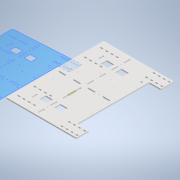
# Autodesk Inventor part: Korpus 3
Saved by Autodesk Inventor 2021.1 (Build 251245010, 245A)
## iProperties
Created: 2023-03-13
Part Number: Korpus 3
Material: Типовые
Document SubType Name: Modeling
Designer: User
Density: 1 g/cm^3
Appearance: По умолчанию
Author: User
Autodesk Inventor part; units mm, degrees
ref_plane "YZ Plane" through (0, 0, 0) normal (1, 0, 0) x (0, 1, 0)
ref_plane "XZ Plane" through (0, 0, 0) normal (0, 1, 0) x (-1, 0, 0)
ref_plane "XY Plane" through (0, 0, 0) normal (0, 0, 1) x (1, 0, 0)
ref_plane "РабПлоскость1" through (117.6762, -49.065, -12.9978) normal (0, -1, 0) x (1, 0, 0)
sketch "Эскиз2" plane through (117.6762, -49.065, -12.9978) normal (0, -1, 0) x (1, 0, 0)
  line L0 (-0.1, 156.35) -> (-0.1, 125.1) projected
  line L1 (-0.1, 125.1) -> (6.1, 125.1) projected
  line L2 (6.1, 156.35) -> (6.1, 125.1) projected
  line L3 (-0.1, 156.35) -> (6.1, 156.35) projected
  line L4 (-0.1, 93.85) -> (-0.1, 62.6) projected
  line L5 (-0.1, 62.6) -> (6.1, 62.6) projected
  line L6 (6.1, 93.85) -> (6.1, 62.6) projected
  line L7 (-0.1, 93.85) -> (6.1, 93.85) projected
  line L8 (-0.1, 31.35) -> (-0.1, 0.1) projected
  line L9 (-0.1, 0.1) -> (6.1, 0.1) projected
  line L10 (6.1, 31.35) -> (6.1, 0.1) projected
  line L11 (-0.1, 31.35) -> (6.1, 31.35) projected
  line L12 (-0.1, -31.15) -> (-0.1, -62.4) projected
  line L13 (-0.1, -62.4) -> (6.1, -62.4) projected
  line L14 (6.1, -31.15) -> (6.1, -62.4) projected
  line L15 (-0.1, -31.15) -> (6.1, -31.15) projected
  line L16 (-0.1, -93.65) -> (-0.1, -124.9) projected
  line L17 (-0.1, -124.9) -> (6.1, -124.9) projected
  line L18 (6.1, -93.65) -> (6.1, -124.9) projected
  line L19 (-0.1, -93.65) -> (6.1, -93.65) projected
  line L20 (-0.1, -156.15) -> (-0.1, -187.4) projected
  line L21 (-0.1, -187.4) -> (6.1, -187.4) projected
  line L22 (6.1, -156.15) -> (6.1, -187.4) projected
  line L23 (-0.1, -156.15) -> (6.1, -156.15) projected
  line L24 (-0.1, -218.65) -> (-0.1, -249.9) projected
  line L25 (-0.1, -249.9) -> (6.1, -249.9) projected
  line L26 (6.1, -218.65) -> (6.1, -249.9) projected
  line L27 (-0.1, -218.65) -> (6.1, -218.65) projected
  line L28 (-0.1, -281.15) -> (-0.1, -312.4) projected
  line L29 (-0.1, -312.4) -> (6.1, -312.4) projected
  line L30 (6.1, -281.15) -> (6.1, -312.4) projected
  line L31 (-0.1, -281.15) -> (6.1, -281.15) projected
  line L32 (21.75, -81.125) -> (59.25, -81.125) projected
  line L33 (59.25, -81.125) -> (59.25, -74.925) projected
  line L34 (21.75, -74.925) -> (59.25, -74.925) projected
  line L35 (21.75, -81.125) -> (21.75, -74.925) projected
  line L36 (96.75, -81.125) -> (134.25, -81.125) projected
  line L37 (134.25, -81.125) -> (134.25, -74.925) projected
  line L38 (96.75, -74.925) -> (134.25, -74.925) projected
  line L39 (96.75, -81.125) -> (96.75, -74.925) projected
  line L40 (-53.25, -81.125) -> (-15.75, -81.125) projected
  line L41 (-15.75, -81.125) -> (-15.75, -74.925) projected
  line L42 (-53.25, -74.925) -> (-15.75, -74.925) projected
  line L43 (-53.25, -81.125) -> (-53.25, -74.925) projected
  line L44 (-128.25, -81.125) -> (-90.75, -81.125) projected
  line L45 (-90.75, -81.125) -> (-90.75, -74.925) projected
  line L46 (-128.25, -74.925) -> (-90.75, -74.925) projected
  line L47 (-128.25, -81.125) -> (-128.25, -74.925) projected
  line L48 (-0.1, -328.025) -> (6.1, -328.025) construction
  line L49 (-147, -81.125) -> (-147, -74.925) construction
  line L50 (-0.1, 171.975) -> (6.1, 171.975) construction
  line L51 (153, -81.125) -> (153, -74.925) construction
  line L52 (208, 171.975) -> (-142, 171.975)
  line L53 (-142, -328.025) -> (208, -328.025)
  line L54 (153, -256.225) -> (153, 100.175)
  line L55 (158, 105.175) -> (208, 105.175)
  line L56 (213, 110.175) -> (213, 166.975)
  line L57 (158, -261.225) -> (208, -261.225)
  line L58 (213, -266.225) -> (213, -323.025)
  arc A0 (213, 166.975) -> (208, 171.975) centre (208, 166.975) ccw
  arc A1 (208, 105.175) -> (213, 110.175) centre (208, 110.175) ccw
  arc A2 (158, 105.175) -> (153, 100.175) centre (158, 100.175) ccw
  arc A3 (153, -256.225) -> (158, -261.225) centre (158, -256.225) ccw
  arc A4 (213, -266.225) -> (208, -261.225) centre (208, -266.225) ccw
  arc A5 (208, -328.025) -> (213, -323.025) centre (208, -323.025) ccw
  line L59 (-147, 166.975) -> (-147, -323.025)
  arc A6 (-142, 171.975) -> (-147, 166.975) centre (-142, 166.975) ccw
  arc A7 (-147, -323.025) -> (-142, -328.025) centre (-142, -323.025) ccw
  point P0 (-117.6762, 12.9978)
  point P1 (153, -78.025)
  point P2 (213, -328.025)
  point P3 (153, -261.225)
  point P4 (-147, -328.025)
  point P5 (-147, 171.975)
  point P6 (153, 105.175)
  point P7 (213, 171.975)
  point P8 (213, 105.175)
  point P9 (213, -261.225)
  point P10 (-147, -78.025)
  point P11 (3, 171.975)
  point P12 (3, -328.025)
  dimension "d5" = 6.2
  dimension "d11" = 60
  dimension "d12" = 66.8
  dimension "d14" = 5
  dimension "d15" = 5
  constraints: 19 point on line, 16 end point, 16 point on circle, 16 tangent, 8 centre point, 6 equal radius, 6 midpoint, 4 perpendicular, 3 horizontal, 1 vertical, 1 vertical alignment
  measures "d5" distance between parallel lines of L34 L32
  measures "d11" distance from line of point (213, 171.975) L54
  measures "d12" distance from line of point (153, 105.175) L52
  measures "d14" radius of A0
  measures "d15" radius of A6
extrude "Корпус" add sketch "Эскиз2" along normal blind 6.2
sketch "Эскиз3" plane through (117.6762, -55.265, -12.9978) normal (0, -1, 0) x (1, 0, 0)
  line L0 (-0.1, -281.15) -> (-0.1, -312.4) construction
  line L1 (-0.1, -312.4) -> (6.1, -312.4) construction
  line L2 (6.1, -281.15) -> (6.1, -312.4) construction
  line L3 (-0.1, -281.15) -> (6.1, -281.15) construction
  line L4 (-0.1, -218.65) -> (-0.1, -249.9) construction
  line L5 (-0.1, -249.9) -> (6.1, -249.9) construction
  line L6 (6.1, -218.65) -> (6.1, -249.9) construction
  line L7 (-0.1, -218.65) -> (6.1, -218.65) construction
  line L8 (-0.1, -156.15) -> (-0.1, -187.4) construction
  line L9 (-0.1, -187.4) -> (6.1, -187.4) construction
  line L10 (6.1, -156.15) -> (6.1, -187.4) construction
  line L11 (-0.1, -156.15) -> (6.1, -156.15) construction
  line L12 (-0.1, -93.65) -> (-0.1, -124.9) construction
  line L13 (-0.1, -124.9) -> (6.1, -124.9) construction
  line L14 (6.1, -93.65) -> (6.1, -124.9) construction
  line L15 (-0.1, -93.65) -> (6.1, -93.65) construction
  line L16 (-0.1, -31.15) -> (-0.1, -62.4) construction
  line L17 (-0.1, -62.4) -> (6.1, -62.4) construction
  line L18 (6.1, -31.15) -> (6.1, -62.4) construction
  line L19 (-0.1, -31.15) -> (6.1, -31.15) construction
  line L20 (-0.1, 31.35) -> (-0.1, 0.1) construction
  line L21 (-0.1, 0.1) -> (6.1, 0.1) construction
  line L22 (6.1, 31.35) -> (6.1, 0.1) construction
  line L23 (-0.1, 31.35) -> (6.1, 31.35) construction
  line L24 (-0.1, 93.85) -> (-0.1, 62.6) construction
  line L25 (-0.1, 62.6) -> (6.1, 62.6) construction
  line L26 (6.1, 93.85) -> (6.1, 62.6) construction
  line L27 (-0.1, 93.85) -> (6.1, 93.85) construction
  line L28 (-0.1, 156.35) -> (-0.1, 125.1) construction
  line L29 (-0.1, 125.1) -> (6.1, 125.1) construction
  line L30 (6.1, 156.35) -> (6.1, 125.1) construction
  line L31 (-0.1, 156.35) -> (6.1, 156.35) construction
  line L32 (21.75, -81.125) -> (59.25, -81.125) construction
  line L33 (59.25, -81.125) -> (59.25, -74.925) construction
  line L34 (21.75, -74.925) -> (59.25, -74.925) construction
  line L35 (21.75, -81.125) -> (21.75, -74.925) construction
  line L36 (96.75, -81.125) -> (134.25, -81.125) construction
  line L37 (134.25, -81.125) -> (134.25, -74.925) construction
  line L38 (96.75, -74.925) -> (134.25, -74.925) construction
  line L39 (96.75, -81.125) -> (96.75, -74.925) construction
  line L40 (-53.25, -81.125) -> (-15.75, -81.125) construction
  line L41 (-15.75, -81.125) -> (-15.75, -74.925) construction
  line L42 (-53.25, -74.925) -> (-15.75, -74.925) construction
  line L43 (-53.25, -81.125) -> (-53.25, -74.925) construction
  line L44 (-128.25, -81.125) -> (-90.75, -81.125) construction
  line L45 (-90.75, -81.125) -> (-90.75, -74.925) construction
  line L46 (-128.25, -74.925) -> (-90.75, -74.925) construction
  line L47 (-128.25, -81.125) -> (-128.25, -74.925) construction
  line L48 (-53.25, -81.125) -> (-90.75, -74.925) construction
  line L49 (96.75, -74.925) -> (134.25, -74.925) construction
  line L50 (59.25, -81.125) -> (96.75, -74.925) construction
  line L51 (6.1, -249.9) -> (-0.1, -249.9) construction
  line L52 (6.1, -281.15) -> (-0.1, -249.9) construction
  line L53 (6.1, -218.65) -> (6.1, -249.9) construction
  line L54 (6.1, -187.4) -> (-0.1, -187.4) construction
  line L55 (6.1, -218.65) -> (-0.1, -187.4) construction
  line L56 (6.1, -156.15) -> (6.1, -187.4) construction
  line L57 (6.1, -156.15) -> (-0.1, -124.9) construction
  line L58 (6.1, -62.4) -> (-0.1, -62.4) construction
  line L59 (6.1, -31.15) -> (6.1, -62.4) construction
  line L60 (6.1, -31.15) -> (-0.1, 0.1) construction
  line L61 (6.1, 31.35) -> (-0.1, 62.6) construction
  line L62 (6.1, 93.85) -> (-0.1, 125.1) construction
  circle A0 centre (3, -265.525) radius 2
  circle A1 centre (3, -140.525) radius 2
  circle A2 centre (3, -15.525) radius 2
  circle A3 centre (3, 109.475) radius 2
  circle A4 centre (-72, -78.025) radius 2
  circle A5 centre (78, -78.025) radius 2
  point P0 (-117.6762, 12.9978)
  dimension "d8" = 4
  constraints: 16 end point, 6 centre point, 6 midpoint, 5 equal radius, 2 parallel
  measures "d8" diameter of A4
extrude "Отверстия" cut sketch "Эскиз3" against normal blind 6.2
sketch "Эскиз6" plane through (117.6762, -55.265, -12.9978) normal (0, -1, 0) x (1, 0, 0)
  line L0 (208, 171.975) -> (-142, 171.975) construction
  line L1 (213, 110.175) -> (213, 166.975) construction
  line L2 (158, 105.175) -> (208, 105.175) construction
  line L3 (-147, 166.975) -> (-147, -323.025) construction
  line L4 (195.1429, 160.775) -> (208, 160.775)
  line L5 (208, 160.775) -> (208, 154.575)
  line L6 (208, 154.575) -> (195.1429, 154.575)
  line L7 (195.1429, 154.575) -> (195.1429, 160.775)
  line L8 (195.1429, 122.575) -> (208, 122.575)
  line L9 (208, 122.575) -> (208, 116.375)
  line L10 (208, 116.375) -> (195.1429, 116.375)
  line L11 (195.1429, 116.375) -> (195.1429, 122.575)
  line L12 (195.1429, 160.775) -> (195.1429, 171.975) construction
  line L13 (195.1429, 116.375) -> (195.1429, 105.175) construction
  line L14 (169.4286, 116.375) -> (169.4286, 122.575)
  line L15 (169.4286, 122.575) -> (182.2857, 122.575)
  line L16 (182.2857, 154.575) -> (169.4286, 154.575)
  line L17 (182.2857, 116.375) -> (169.4286, 116.375)
  line L18 (182.2857, 160.775) -> (182.2857, 154.575)
  line L19 (169.4286, 154.575) -> (169.4286, 160.775)
  line L20 (169.4286, 160.775) -> (182.2857, 160.775)
  line L21 (182.2857, 122.575) -> (182.2857, 116.375)
  line L22 (143.7143, 116.375) -> (143.7143, 122.575)
  line L23 (143.7143, 122.575) -> (156.5714, 122.575)
  line L24 (156.5714, 154.575) -> (143.7143, 154.575)
  line L25 (156.5714, 116.375) -> (143.7143, 116.375)
  line L26 (156.5714, 160.775) -> (156.5714, 154.575)
  line L27 (143.7143, 154.575) -> (143.7143, 160.775)
  line L28 (143.7143, 160.775) -> (156.5714, 160.775)
  line L29 (156.5714, 122.575) -> (156.5714, 116.375)
  line L30 (118, 116.375) -> (118, 122.575)
  line L31 (118, 122.575) -> (130.8571, 122.575)
  line L32 (130.8571, 154.575) -> (118, 154.575)
  line L33 (130.8571, 116.375) -> (118, 116.375)
  line L34 (130.8571, 160.775) -> (130.8571, 154.575)
  line L35 (118, 154.575) -> (118, 160.775)
  line L36 (118, 160.775) -> (130.8571, 160.775)
  line L37 (130.8571, 122.575) -> (130.8571, 116.375)
  line L38 (0, 93.85) -> (0, 62.6) construction
  line L39 (-0.1, 62.5) -> (6.1, 62.5) construction
  line L40 (6, 93.85) -> (6, 62.6) construction
  line L41 (-0.1, 93.75) -> (6.1, 93.75) construction
  line L42 (-53.25, -81.125) -> (-15.75, -81.125) construction
  line L43 (-15.75, -81.125) -> (-15.75, -74.925) construction
  line L44 (-53.25, -74.925) -> (-15.75, -74.925) construction
  line L45 (-53.25, -81.125) -> (-53.25, -74.925) construction
  line L46 (21.75, -81.125) -> (59.25, -81.125) construction
  line L47 (59.25, -81.125) -> (59.25, -74.925) construction
  line L48 (21.75, -74.925) -> (59.25, -74.925) construction
  line L49 (21.75, -81.125) -> (21.75, -74.925) construction
  line L50 (-15.75, -78.025) -> (21.75, -78.025) construction
  line L51 (-127, 137.075) -> (-113.7143, 137.075)
  line L52 (-113.7143, 137.075) -> (-113.7143, 130.875)
  line L53 (-113.7143, 130.875) -> (-127, 130.875)
  line L54 (-127, 130.875) -> (-127, 137.075)
  line L55 (-127, 54.075) -> (-113.7143, 54.075)
  line L56 (-113.7143, 54.075) -> (-113.7143, 47.875)
  line L57 (-113.7143, 47.875) -> (-127, 47.875)
  line L58 (-127, 47.875) -> (-127, 54.075)
  line L59 (-100.4286, 54.075) -> (-87.1429, 54.075)
  line L60 (-87.1429, 47.875) -> (-100.4286, 47.875)
  line L61 (-100.4286, 47.875) -> (-100.4286, 54.075)
  line L62 (-87.1429, 137.075) -> (-87.1429, 130.875)
  line L63 (-87.1429, 130.875) -> (-100.4286, 130.875)
  line L64 (-100.4286, 137.075) -> (-87.1429, 137.075)
  line L65 (-100.4286, 130.875) -> (-100.4286, 137.075)
  line L66 (-87.1429, 54.075) -> (-87.1429, 47.875)
  line L67 (-73.8571, 54.075) -> (-60.5714, 54.075)
  line L68 (-60.5714, 47.875) -> (-73.8571, 47.875)
  line L69 (-73.8571, 47.875) -> (-73.8571, 54.075)
  line L70 (-60.5714, 137.075) -> (-60.5714, 130.875)
  line L71 (-60.5714, 130.875) -> (-73.8571, 130.875)
  line L72 (-73.8571, 137.075) -> (-60.5714, 137.075)
  line L73 (-73.8571, 130.875) -> (-73.8571, 137.075)
  line L74 (-60.5714, 54.075) -> (-60.5714, 47.875)
  line L75 (-47.2857, 54.075) -> (-34, 54.075)
  line L76 (-34, 47.875) -> (-47.2857, 47.875)
  line L77 (-47.2857, 47.875) -> (-47.2857, 54.075)
  line L78 (-34, 137.075) -> (-34, 130.875)
  line L79 (-34, 130.875) -> (-47.2857, 130.875)
  line L80 (-47.2857, 137.075) -> (-34, 137.075)
  line L81 (-47.2857, 130.875) -> (-47.2857, 137.075)
  line L82 (-34, 54.075) -> (-34, 47.875)
  line L83 (-15.75, 93.85) -> (-53.25, 93.85)
  line L84 (-53.25, 93.85) -> (-53.25, 62.6)
  line L85 (-53.25, 62.6) -> (-15.75, 62.6)
  line L86 (-15.75, 62.6) -> (-15.75, 93.85)
  line L87 (21.75, 62.6) -> (59.25, 62.6)
  line L88 (59.25, 62.6) -> (59.25, 93.85)
  line L89 (59.25, 93.85) -> (21.75, 93.85)
  line L90 (21.75, 93.85) -> (21.75, 62.6)
  line L91 (-113.7143, 130.875) -> (-100.4286, 137.075) construction
  line L92 (-60.5714, 130.875) -> (-47.2857, 137.075) construction
  line L93 (-113.7143, 47.875) -> (-100.4286, 54.075) construction
  line L94 (-60.5714, 47.875) -> (-47.2857, 54.075) construction
  line L95 (130.8571, 154.575) -> (143.7143, 160.775) construction
  line L96 (182.2857, 154.575) -> (195.1429, 160.775) construction
  line L97 (130.8571, 116.375) -> (143.7143, 122.575) construction
  line L98 (182.2857, 116.375) -> (195.1429, 122.575) construction
  circle A0 centre (-107.0714, 133.975) radius 1.5
  circle A1 centre (-53.9286, 133.975) radius 1.5
  circle A2 centre (-107.0714, 50.975) radius 1.5
  circle A3 centre (-53.9286, 50.975) radius 1.5
  circle A4 centre (137.2857, 157.675) radius 1.5
  circle A5 centre (188.7143, 157.675) radius 1.5
  circle A6 centre (188.7143, 119.475) radius 1.5
  circle A7 centre (137.2857, 119.475) radius 1.5
  line L99 (195.1429, -316.825) -> (208, -316.825)
  line L100 (208, -316.825) -> (208, -310.625)
  line L101 (208, -310.625) -> (195.1429, -310.625)
  line L102 (195.1429, -310.625) -> (195.1429, -316.825)
  line L103 (195.1429, -278.625) -> (208, -278.625)
  line L104 (208, -278.625) -> (208, -272.425)
  line L105 (208, -272.425) -> (195.1429, -272.425)
  line L106 (195.1429, -272.425) -> (195.1429, -278.625)
  line L107 (195.1429, -316.825) -> (195.1429, -328.025) construction
  line L108 (169.4286, -272.425) -> (169.4286, -278.625)
  line L109 (169.4286, -278.625) -> (182.2857, -278.625)
  line L110 (182.2857, -310.625) -> (169.4286, -310.625)
  line L111 (182.2857, -272.425) -> (169.4286, -272.425)
  line L112 (182.2857, -316.825) -> (182.2857, -310.625)
  line L113 (169.4286, -310.625) -> (169.4286, -316.825)
  line L114 (169.4286, -316.825) -> (182.2857, -316.825)
  line L115 (182.2857, -278.625) -> (182.2857, -272.425)
  line L116 (143.7143, -272.425) -> (143.7143, -278.625)
  line L117 (143.7143, -278.625) -> (156.5714, -278.625)
  line L118 (156.5714, -310.625) -> (143.7143, -310.625)
  line L119 (156.5714, -272.425) -> (143.7143, -272.425)
  line L120 (156.5714, -316.825) -> (156.5714, -310.625)
  line L121 (143.7143, -310.625) -> (143.7143, -316.825)
  line L122 (143.7143, -316.825) -> (156.5714, -316.825)
  line L123 (156.5714, -278.625) -> (156.5714, -272.425)
  line L124 (118, -272.425) -> (118, -278.625)
  line L125 (118, -278.625) -> (130.8571, -278.625)
  line L126 (130.8571, -310.625) -> (118, -310.625)
  line L127 (130.8571, -272.425) -> (118, -272.425)
  line L128 (130.8571, -316.825) -> (130.8571, -310.625)
  line L129 (118, -310.625) -> (118, -316.825)
  line L130 (118, -316.825) -> (130.8571, -316.825)
  line L131 (130.8571, -278.625) -> (130.8571, -272.425)
  line L132 (130.8571, -310.625) -> (143.7143, -316.825) construction
  line L133 (182.2857, -310.625) -> (195.1429, -316.825) construction
  line L134 (130.8571, -272.425) -> (143.7143, -278.625) construction
  line L135 (182.2857, -272.425) -> (195.1429, -278.625) construction
  circle A8 centre (137.2857, -313.725) radius 1.5
  circle A9 centre (188.7143, -313.725) radius 1.5
  circle A10 centre (188.7143, -275.525) radius 1.5
  circle A11 centre (137.2857, -275.525) radius 1.5
  line L136 (-147, -323.025) -> (-147, 166.975) construction
  line L137 (-127, -293.125) -> (-113.7143, -293.125)
  line L138 (-113.7143, -293.125) -> (-113.7143, -286.925)
  line L139 (-113.7143, -286.925) -> (-127, -286.925)
  line L140 (-127, -286.925) -> (-127, -293.125)
  line L141 (-127, -210.125) -> (-113.7143, -210.125)
  line L142 (-113.7143, -210.125) -> (-113.7143, -203.925)
  line L143 (-113.7143, -203.925) -> (-127, -203.925)
  line L144 (-127, -203.925) -> (-127, -210.125)
  line L145 (-100.4286, -210.125) -> (-87.1429, -210.125)
  line L146 (-87.1429, -203.925) -> (-100.4286, -203.925)
  line L147 (-100.4286, -203.925) -> (-100.4286, -210.125)
  line L148 (-87.1429, -293.125) -> (-87.1429, -286.925)
  line L149 (-87.1429, -286.925) -> (-100.4286, -286.925)
  line L150 (-100.4286, -293.125) -> (-87.1429, -293.125)
  line L151 (-100.4286, -286.925) -> (-100.4286, -293.125)
  line L152 (-87.1429, -210.125) -> (-87.1429, -203.925)
  line L153 (-73.8571, -210.125) -> (-60.5714, -210.125)
  line L154 (-60.5714, -203.925) -> (-73.8571, -203.925)
  line L155 (-73.8571, -203.925) -> (-73.8571, -210.125)
  line L156 (-60.5714, -293.125) -> (-60.5714, -286.925)
  line L157 (-60.5714, -286.925) -> (-73.8571, -286.925)
  line L158 (-73.8571, -293.125) -> (-60.5714, -293.125)
  line L159 (-73.8571, -286.925) -> (-73.8571, -293.125)
  line L160 (-60.5714, -210.125) -> (-60.5714, -203.925)
  line L161 (-47.2857, -210.125) -> (-34, -210.125)
  line L162 (-34, -203.925) -> (-47.2857, -203.925)
  line L163 (-47.2857, -203.925) -> (-47.2857, -210.125)
  line L164 (-34, -293.125) -> (-34, -286.925)
  line L165 (-34, -286.925) -> (-47.2857, -286.925)
  line L166 (-47.2857, -293.125) -> (-34, -293.125)
  line L167 (-47.2857, -286.925) -> (-47.2857, -293.125)
  line L168 (-34, -210.125) -> (-34, -203.925)
  line L169 (-15.75, -249.9) -> (-53.25, -249.9)
  line L170 (-53.25, -249.9) -> (-53.25, -218.65)
  line L171 (-53.25, -218.65) -> (-15.75, -218.65)
  line L172 (-15.75, -218.65) -> (-15.75, -249.9)
  line L173 (-113.7143, -286.925) -> (-100.4286, -293.125) construction
  line L174 (-60.5714, -286.925) -> (-47.2857, -293.125) construction
  line L175 (-113.7143, -203.925) -> (-100.4286, -210.125) construction
  line L176 (-60.5714, -203.925) -> (-47.2857, -210.125) construction
  circle A12 centre (-107.0714, -290.025) radius 1.5
  circle A13 centre (-53.9286, -290.025) radius 1.5
  circle A14 centre (-107.0714, -207.025) radius 1.5
  circle A15 centre (-53.9286, -207.025) radius 1.5
  line L177 (21.75, -218.65) -> (59.25, -218.65)
  line L178 (59.25, -218.65) -> (59.25, -249.9)
  line L179 (59.25, -249.9) -> (21.75, -249.9)
  line L180 (21.75, -249.9) -> (21.75, -218.65)
  line L181 (208, -261.225) -> (158, -261.225) construction
  line L182 (153, -256.225) -> (153, 100.175) construction
  circle A16 centre (133, -241.225) radius 5.75
  line L183 (-127, 130.875) -> (-34, 54.075) construction
  line L184 (-100.4286, 130.875) -> (-100.4286, 105.275) construction
  point P0 (-117.6762, 12.9978)
  point P1 (-0.1, 93.85)
  point P2 (-0.1, 62.6)
  point P3 (6.1, 62.6)
  point P4 (6.1, 93.85)
  dimension "d72" = 5
  dimension "d73" = 12.8571
  dimension "d74" = 6.2
  dimension "d75" = 11.2
  dimension "d78" = 25.7143
  dimension "d83" = 13.2857
  dimension "d84" = 6.2
  dimension "d86" = 34.9
  dimension "d87" = 20
  dimension "d90" = 26.5714
  dimension "d95" = 3
  dimension "d96" = 11.5
  dimension "d97" = 20
  dimension "d98" = 20
  dimension "d104" = 89.2
  dimension "d105" = 76.8
  dimension "d110" = 25.6
  constraints: 334 end point, 83 symmetric about line, 17 centre point, 17 parallel, 10 midpoint, 8 horizontal, 8 vertical alignment, 7 equal radius, 7 perpendicular, 4 horizontal alignment, 3 collinear, 3 point on line, 1 vertical, 104 other
  measures "d72" distance between parallel lines of L1 L5
  measures "d73" distance of L5.end L6.end
  measures "d74" distance of L6.end L4.start
  measures "d75" distance between parallel lines of L0 L4
  measures "d78" distance of L10.end L14.start
  measures "d83" distance of L51.start L51.end
  measures "d84" distance of L53.end L51.start
  measures "d86" distance between parallel lines of L0 L51
  measures "d87" distance between parallel lines of L3 L54
  measures "d90" distance of L55.end L59.end
  measures "d95" diameter of A7
  measures "d96" diameter of A16
  measures "d97" distance from line of L182 A16.centre
  measures "d98" distance from line of A16.centre L181
  measures "d104" distance between parallel lines of L76 L80
  measures "d105" distance between parallel lines of L55 L53
  measures "d110" distance of L63.end L184.end
extrude "Выдавливание5" cut sketch "Эскиз6" against normal blind 6.2
sketch "Эскиз7" plane through (117.6762, -55.265, -12.9978) normal (0, -1, 0) x (1, 0, 0)
  line L0 (-100.4286, 137.075) -> (-87.1429, 137.075) construction
  line L1 (-87.1429, 137.075) -> (-87.1429, 130.875) construction
  line L2 (-100.4286, 130.875) -> (-87.1429, 130.875) construction
  line L3 (-100.4286, 137.075) -> (-100.4286, 130.875) construction
  line L4 (-60.5714, 54.075) -> (-60.5714, 47.875) construction
  line L5 (-60.5714, 47.875) -> (-73.8571, 47.875) construction
  line L6 (-73.8571, 47.875) -> (-73.8571, 54.075) construction
  line L7 (-73.8571, 54.075) -> (-60.5714, 54.075) construction
  line L8 (-87.1429, 130.875) -> (-73.8571, 54.075) construction
  line L9 (-83.6, 105.275) -> (-77.4, 105.275)
  line L10 (-77.4, 105.275) -> (-77.4, 79.675)
  line L11 (-77.4, 79.675) -> (-83.6, 79.675)
  line L12 (-83.6, 79.675) -> (-83.6, 105.275)
  line L13 (-83.6, 105.275) -> (-77.4, 79.675) construction
  line L14 (-77.4, 105.275) -> (-83.6, 79.675) construction
  line L15 (-53.25, -81.125) -> (-15.75, -81.125) construction
  line L16 (-15.75, -81.125) -> (-15.75, -74.925) construction
  line L17 (-53.25, -74.925) -> (-15.75, -74.925) construction
  line L18 (-53.25, -81.125) -> (-53.25, -74.925) construction
  line L19 (21.75, -81.125) -> (59.25, -81.125) construction
  line L20 (59.25, -81.125) -> (59.25, -74.925) construction
  line L21 (21.75, -74.925) -> (59.25, -74.925) construction
  line L22 (21.75, -81.125) -> (21.75, -74.925) construction
  line L23 (21.75, -81.125) -> (21.75, -74.925) projected
  line L24 (21.75, -78.025) -> (-15.75, -78.025) construction
  line L25 (-83.6, -261.325) -> (-77.4, -261.325)
  line L26 (-77.4, -261.325) -> (-77.4, -235.725)
  line L27 (-77.4, -235.725) -> (-83.6, -235.725)
  line L28 (-83.6, -235.725) -> (-83.6, -261.325)
  line L29 (-83.6, -261.325) -> (-77.4, -235.725) construction
  line L30 (-77.4, -261.325) -> (-83.6, -235.725) construction
  point P0 (-117.6762, 12.9978)
  point P1 (-80.5, 92.475)
  point P2 (-80.5, 92.475)
  point P3 (-80.5, -248.525)
  point P4 (-80.5, -248.525)
  dimension "d111" = 25.6
  dimension "d112" = 6.2
  constraints: 28 end point, 8 midpoint, 6 symmetric about line, 2 parallel, 1 horizontal, 1 perpendicular
  measures "d111" distance of L9.end L10.end
  measures "d112" distance of L10.end L11.end
extrude "Выдавливание6" cut sketch "Эскиз7" against normal blind 6.2
sketch "Эскиз8" plane through (117.6762, -49.065, -12.9978) normal (0, 1, 0) x (1, 0, 0)
  point P0 (-117.6762, -12.9978)
sketch "Эскиз9" plane through (117.6762, -55.265, -12.9978) normal (0, -1, 0) x (1, 0, 0)
  circle A0 centre (-141, -28.768) radius 1.6 projected
  circle A1 centre (-141, -123.768) radius 1.6 projected
  circle A2 centre (-108, -123.768) radius 1.6 projected
  circle A3 centre (-108, -28.768) radius 1.6 projected
  circle A4 centre (-75.5, -28.768) radius 1.6 projected
  circle A5 centre (-75.5, -123.768) radius 1.6 projected
  circle A6 centre (-32.75, -108.518) radius 1.6 projected
  circle A7 centre (-9, -174.776) radius 1.5 projected
  circle A8 centre (-9, -65.2685) radius 1.5 projected
  circle A9 centre (-9, 44.239) radius 1.5 projected
  circle A10 centre (42.8781, 44.239) radius 1.5 projected
  circle A11 centre (81, 21.888) radius 1.5 projected
  circle A12 centre (143, 21.888) radius 1.5 projected
  circle A13 centre (143, -65.2685) radius 1.5 projected
  circle A14 centre (143, -152.425) radius 1.5 projected
  circle A15 centre (81, -152.425) radius 1.5 projected
  circle A16 centre (42.8781, -174.776) radius 1.5 projected
  circle A17 centre (67, -65.2685) radius 1.5 projected
  point P0 (-117.6762, 12.9978)
extrude "Выдавливание7" cut sketch "Эскиз9" against normal blind 6.2 contours A0 | A1 | A2 | A3 | A4 | A5 | A6 | A7 | A9 | A10 | A11 | A12 | A13 | A14 | A15 | A16 | A17
equation "\"d6\" = d5"
equation "\"d9\" = d5"
